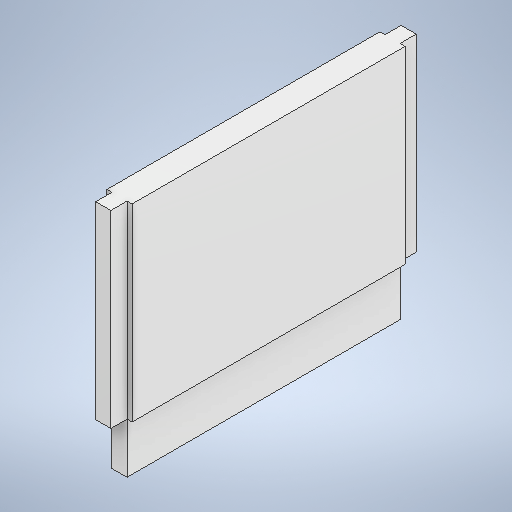
# Autodesk Inventor part: sciana_bezdziury
Saved by Autodesk Inventor 2025.2 (Build 292293000, 293)
## iProperties
Created: 2026-07-07
Part Number: sciana_bezdziury
Material: ABS Plastic
Document SubType Name: Modeling
Designer: ksawe
Density: 1.06 g/cm^3
Appearance: Smooth - White
Author: ksawe
Autodesk Inventor part; units mm, degrees
ref_plane "YZ Plane" through (0, 0, 0) normal (1, 0, 0) x (0, 1, 0)
ref_plane "XZ Plane" through (0, 0, 0) normal (0, 1, 0) x (-1, 0, 0)
ref_plane "XY Plane" through (0, 0, 0) normal (0, 0, 1) x (1, 0, 0)
sketch "Sketch1" plane through (0, 0, 0) normal (0, 1, 0) x (-1, 0, 0)
  point P0 (0, 0)
sketch "Sketch2" plane through (0, 0, 0) normal (0, 1, 0) x (-1, 0, 0)
  line L0 (5, 54.202) -> (-5, 54.202)
  line L1 (-5, 54.202) -> (-5, -54.202)
  line L2 (-5, -54.202) -> (5, -54.202)
  line L3 (5, -54.202) -> (5, 54.202)
  line L4 (5, 54.202) -> (-5, -54.202) construction
  line L5 (-5, 54.202) -> (5, -54.202) construction
  line L6 (3, 60.655) -> (-3, 60.655)
  line L7 (-3, 60.655) -> (-3, -60.655)
  line L8 (-3, -60.655) -> (3, -60.655)
  line L9 (3, -60.655) -> (3, 60.655)
  line L10 (3, 60.655) -> (-3, -60.655) construction
  line L11 (-3, 60.655) -> (3, -60.655) construction
  point P0 (0, 0)
  point P1 (3, 54.202)
  point P2 (-3, 54.202)
  point P3 (-3, -54.202)
  point P4 (3, -54.202)
  dimension "d0" = 10
  dimension "d1" = 108.404
  dimension "d2" = 6
  dimension "d3" = 121.31
  constraints: 24 end point, 4 midpoint, 4 parallel, 2 horizontal, 2 perpendicular
  measures "d0" distance between parallel lines of L1 L3
  measures "d1" distance between parallel lines of L2 L0
  measures "d2" distance of L8.end L7.end
  measures "d3" distance of L7.end L6.end
extrude "Extrusion1" add sketch "Sketch2" along normal blind 75
extrude "Extrusion2" add sketch "Sketch2" against normal blind 20 contours L9 L2 L7 L0
body "Solid1"
